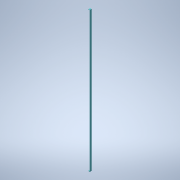
# Autodesk Inventor part: CHAPA_UNIAO_ROLAMENTOS
Saved by Autodesk Inventor 2020 (Build 240168000, 168)
## iProperties
Created: 2016-03-03
Part Number: CHAPA_UNIAO_ROLAMENTOS
Material: Genérico
Document SubType Name: Modeling
Designer: Everton
Density: 1 g/cm^3
Appearance: Padrão
Author: Everton
Autodesk Inventor part; units mm, degrees
ref_plane "YZ Plane" through (0, 0, 0) normal (1, 0, 0) x (0, 1, 0)
ref_plane "XZ Plane" through (0, 0, 0) normal (0, 1, 0) x (-1, 0, 0)
ref_plane "XY Plane" through (0, 0, 0) normal (0, 0, 1) x (1, 0, 0)
sketch "Sketch1" plane through (0, 0, 0) normal (0, 1, 0) x (-1, 0, 0)
  line L0 (7.6961, -19.417) -> (7.6961, -1319.417)
  line L1 (7.6961, -1319.417) -> (17.6961, -1319.417)
  line L2 (7.6961, -19.417) -> (17.6961, -19.417)
  line L3 (20.8711, -22.592) -> (10.8711, -22.592)
  line L4 (10.8711, -22.592) -> (10.8711, -1316.242)
  line L5 (10.8711, -1316.242) -> (20.8711, -1316.242)
  line L6 (20.8711, -22.592) -> (20.8711, -19.417)
  line L7 (20.8711, -19.417) -> (17.6961, -19.417)
  line L8 (20.8711, -1316.242) -> (20.8711, -1319.417)
  line L9 (20.8711, -1319.417) -> (17.6961, -1319.417)
  point P0 (0, 0)
  dimension "d0" = 1300
  dimension "d1" = 10
  dimension "d4" = 10
  dimension "d5" = 10
  constraints: 20 end point, 4 perpendicular, 3 vertical, 1 horizontal, 2 other
  measures "d0" distance of L0.start L0.end
  measures "d1" distance of L0.end L1.end
  measures "d4" distance of L3.end L3.start
  measures "d5" distance of L4.end L5.end
extrude "Extrusion1" add sketch "Sketch1" along normal blind 16
body "Solid1"
